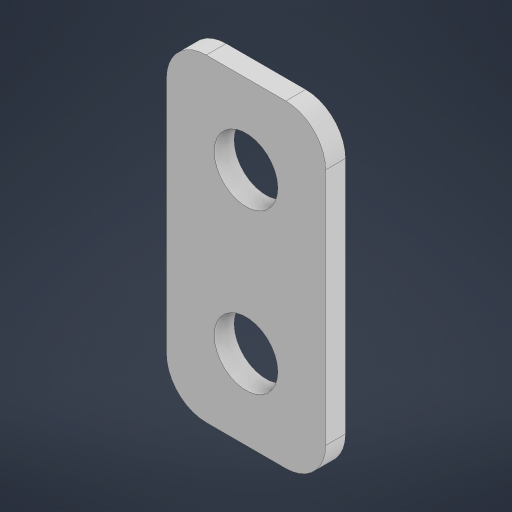
# Autodesk Inventor part: polySpacer2
Saved by Autodesk Inventor 2023.4 (Build 274418000, 418)
## iProperties
Created: 2024-03-08
Part Number: polySpacer2
Material: Generic
Document SubType Name: Modeling
Designer: Meer
Density: 1 g/cm^3
Appearance: Default
Author: Meer
Autodesk Inventor part; units mm, degrees
ref_plane "YZ Plane" through (0, 0, 0) normal (1, 0, 0) x (0, 1, 0)
ref_plane "XZ Plane" through (0, 0, 0) normal (0, 1, 0) x (-1, 0, 0)
ref_plane "XY Plane" through (0, 0, 0) normal (0, 0, 1) x (1, 0, 0)
sketch "Sketch1" plane through (0, 0, 0) normal (0, 0, 1) x (1, 0, 0)
  line L0 (0, 0) -> (12.7, 0)
  line L1 (12.7, 0) -> (12.7, 25.4)
  line L2 (12.7, 25.4) -> (0, 25.4)
  line L3 (0, 25.4) -> (0, 0)
  line L4 (6.35, 0) -> (6.35, 6.35)
  circle A0 centre (6.35, 6.35) radius 2.54
  line L5 (6.35, 6.35) -> (6.35, 19.05)
  circle A1 centre (6.35, 19.05) radius 2.54
  dimension "d0" = 12.7
  dimension "d1" = 25.4
  dimension "d2" = 6.35
  dimension "d3" = 5.08
  dimension "d4" = 12.7
  dimension "d5" = 5.08
  constraints: 12 end point, 2 centre point, 2 coincident, 2 parallel, 2 vertical, 1 horizontal, 1 midpoint, 1 perpendicular
  measures "d0" distance of L2.end L1.end
  measures "d1" distance of L0.end L1.end
  measures "d2" distance of L4.start L4.end
  measures "d3" diameter of A0
  measures "d4" distance of L5.start L5.end
  measures "d5" diameter of A1
extrude "Extrusion1" add sketch "Sketch1" along normal blind 1.5875
fillet "Fillet1" radius 3.175 4 edges at (12.7, 25.4, 0.7937) (0, 25.4, 0.7937) (12.7, 0, 0.7937) (0, 0, 0.7937)
body "Solid1"
